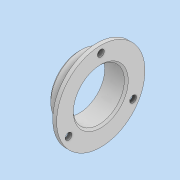
# Autodesk Inventor part: Deckel oben
Saved by Autodesk Inventor 2021 (Build 250183000, 183)
## iProperties
Created: 2024-03-13
Part Number: Deckel oben
Material: Generic
Document SubType Name: Modeling
Designer: Nokia
Density: 1 g/cm^3
Appearance: Default
Author: Nokia
Autodesk Inventor part; units mm, degrees
ref_plane "YZ Plane" through (0, 0, 0) normal (1, 0, 0) x (0, 1, 0)
ref_plane "XZ Plane" through (0, 0, 0) normal (0, 1, 0) x (-1, 0, 0)
ref_plane "XY Plane" through (0, 0, 0) normal (0, 0, 1) x (1, 0, 0)
sketch "Sketch1" plane through (0, 0, 0) normal (0, 0, 1) x (1, 0, 0)
  line L0 (0, 26) -> (-18, 26)
  line L1 (-18, 26) -> (-18, 31)
  line L2 (-18, 31) -> (0, 31)
  line L3 (0, 31) -> (0, 45)
  line L4 (0, 45) -> (4, 45)
  line L5 (4, 45) -> (4, 26)
  line L6 (4, 26) -> (0, 26)
  line L7 (29.142, 0) -> (-45.5287, 0)
  point P0 (0, 0)
  dimension "d0" = 26
  dimension "d1" = 18
  dimension "d2" = 5
  dimension "d3" = 14
  dimension "d4" = 4
  constraints: 16 end point, 5 perpendicular, 3 horizontal
  measures "d0" distance of point (0, 0) L0.start
  measures "d1" distance of L0.start L0.end
  measures "d2" distance of L0.end L1.end
  measures "d3" distance of L2.end L3.end
  measures "d4" distance of L3.end L4.end
revolve "Revolution1" add sketch "Sketch1" angle 360 about axis through (29.142, 0, 0) along (-1, 0, 0)
sketch "Sketch2" plane through (4, 0, 0) normal (1, 0, 0) x (0, 0, -1)
  circle A0 centre (0, 0) radius 45 projected
  line L0 (0, 45) -> (0, 38)
  circle A1 centre (0, 38) radius 3.5
  dimension "d6" = 7
  constraints: 2 end point, 1 centre point, 1 coincident, 1 vertical, 1 vertical alignment, 1 other
  measures "d6" distance of L0.start L0.end
hole "Hole1" at (4, 38, 0) direction (-1, 0, 0) diameter 7 end through all
pattern_circular "Circular Pattern1" count 3 over 360 about axis through (-10, 0, 0) along (1, 0, 0) of "Hole1"
chamfer "Chamfer1" distance 2 angle 45 2 edges at (-18, -31, 0) (4, -26, 0)
body "Solid1"
